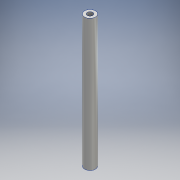
# Autodesk Inventor part: スペーサーm3-73　簡易筒型
Saved by Autodesk Inventor 2016 (Build 200138000, 138)
## iProperties
Created: 2016-02-18
Part Number: スペーサーm3-73　簡易筒型
Material: アルミニウム 2014-T4
Document SubType Name: Modeling
Designer: Takumi
Density: 2.8 g/cm^3
Appearance: アルミニウム - フラット
Mass: 5.52891 g
Surface Area: 26.9806 cm^2
Volume: 1.97461 cm^3
Author: Takumi
Autodesk Inventor part; units mm, degrees
ref_plane "YZ Plane" through (0, 0, 0) normal (1, 0, 0) x (0, 1, 0)
ref_plane "XZ Plane" through (0, 0, 0) normal (0, 1, 0) x (-1, 0, 0)
ref_plane "XY Plane" through (0, 0, 0) normal (0, 0, 1) x (1, 0, 0)
sketch "スケッチ1" plane through (0, 0, 0) normal (0, 0, 1) x (1, 0, 0)
  circle A0 centre (0, 0) radius 3
  circle A1 centre (0, 0) radius 1.5005
  dimension "d0" = 6
  dimension "d1" = 3.001
  constraints: 2 centre point, 2 coincident
  measures "d0" diameter of A0
  measures "d1" diameter of A1
extrude "押し出し1" add sketch "スケッチ1" along normal blind 73
sketch "スケッチ2" plane through (0, 0, 73) normal (0, 0, 1) x (1, 0, 0)
  circle A0 centre (0, 0) radius 1.5005 projected
  circle A1 centre (0, 0) radius 1.5
  dimension "d4" = 3
  constraints: 1 centre point, 1 coincident
  measures "d4" diameter of A1
extrude "押し出し2" add sketch "スケッチ2" against normal blind 73
hole "穴1" at (0, 0, 73) direction (0, 0, -1) diameter 3 depth 6 tip angle 118
hole "穴2" at (0, 0, 0) direction (0, 0, 1) diameter 3 depth 6 tip angle 118
